Autodesk Inventor part; units mm, degrees
(part 3 of 6)
  line L900 (29.3831, -15.4753) -> (29.375, -15.3073) construction
  line L901 (29.375, -15.3073) -> (29.4167, -15.1213) construction
  line L902 (29.4167, -15.1213) -> (29.4167, -15.1153)
  spline S269 degree 3 poles (29.4167, -15.1153) (29.4167, -15.1093) (29.4252, -15.1093) (29.4252, -15.1034) knots 10 10 10 10 11 11 11 11
  line L903 (29.4167, -15.1153) -> (29.4167, -15.1093) construction
  line L904 (29.4167, -15.1093) -> (29.4252, -15.1093) construction
  line L905 (29.4252, -15.1093) -> (29.4252, -15.1034) construction
  line L906 (29.4252, -15.1034) -> (29.4149, -15.1093)
  spline S270 degree 3 poles (29.4149, -15.1093) (29.4209, -15.1034) (29.4167, -15.1034) (29.4167, -15.0974) knots 12 12 12 12 13 13 13 13
  line L907 (29.4149, -15.1093) -> (29.4209, -15.1034) construction
  line L908 (29.4209, -15.1034) -> (29.4167, -15.1034) construction
  line L909 (29.4167, -15.1034) -> (29.4167, -15.0974) construction
  line L910 (29.4167, -15.0974) -> (29.4167, -15.0673)
  spline S271 degree 3 poles (29.4167, -15.0673) (29.5, -14.7134) (29.6142, -14.3654) (29.7402, -14.0234) knots 14 14 14 14 15 15 15 15
  line L911 (29.4167, -15.0673) -> (29.5, -14.7134) construction
  line L912 (29.5, -14.7134) -> (29.6142, -14.3654) construction
  line L913 (29.6142, -14.3654) -> (29.7402, -14.0234) construction
  spline S272 degree 3 poles (29.7402, -14.0234) (29.8722, -13.6634) (30.0009, -13.3094) (30.1689, -12.9674) knots 15 15 15 15 16 16 16 16
  line L914 (29.7402, -14.0234) -> (29.8722, -13.6634) construction
  line L915 (29.8722, -13.6634) -> (30.0009, -13.3094) construction
  line L916 (30.0009, -13.3094) -> (30.1689, -12.9674) construction
  spline S273 degree 3 poles (30.1689, -12.9674) (30.3249, -12.6434) (30.5063, -12.3254) (30.7103, -12.0314) knots 16 16 16 16 17 17 17 17
  line L917 (30.1689, -12.9674) -> (30.3249, -12.6434) construction
  line L918 (30.3249, -12.6434) -> (30.5063, -12.3254) construction
  line L919 (30.5063, -12.3254) -> (30.7103, -12.0314) construction
  spline S274 degree 3 poles (30.7103, -12.0314) (30.8903, -11.7614) (31.1069, -11.4674) (31.3829, -11.2874) knots 17 17 17 17 18 18 18 18
  line L920 (30.7103, -12.0314) -> (30.8903, -11.7614) construction
  line L921 (30.8903, -11.7614) -> (31.1069, -11.4674) construction
  line L922 (31.1069, -11.4674) -> (31.3829, -11.2874) construction
  spline S275 degree 3 poles (31.3829, -11.2874) (31.467, -11.2634) (31.5513, -11.1734) (31.6593, -11.1914) knots 18 18 18 18 19 19 19 19
  line L923 (31.3829, -11.2874) -> (31.467, -11.2634) construction
  line L924 (31.467, -11.2634) -> (31.5513, -11.1734) construction
  line L925 (31.5513, -11.1734) -> (31.6593, -11.1914) construction
  spline S276 degree 3 poles (31.6593, -11.1914) (31.7673, -11.2094) (31.7675, -11.3234) (31.7435, -11.4314) knots 19 19 19 19 20 20 20 20
  line L926 (31.6593, -11.1914) -> (31.7673, -11.2094) construction
  line L927 (31.7673, -11.2094) -> (31.7675, -11.3234) construction
  line L928 (31.7675, -11.3234) -> (31.7435, -11.4314) construction
  spline S277 degree 3 poles (31.7435, -11.4314) (31.7735, -11.3474) (31.7915, -11.2574) (31.7196, -11.1974) knots 20 20 20 20 21 21 21 21
  line L929 (31.7435, -11.4314) -> (31.7735, -11.3474) construction
  line L930 (31.7735, -11.3474) -> (31.7915, -11.2574) construction
  line L931 (31.7915, -11.2574) -> (31.7196, -11.1974) construction
  spline S278 degree 3 poles (31.7196, -11.1974) (31.6235, -11.1254) (31.4376, -11.2394) (31.3596, -11.2934) knots 21 21 21 21 22 22 22 22
  line L932 (31.7196, -11.1974) -> (31.6235, -11.1254) construction
  line L933 (31.6235, -11.1254) -> (31.4376, -11.2394) construction
  line L934 (31.4376, -11.2394) -> (31.3596, -11.2934) construction
  spline S279 degree 3 poles (31.3596, -11.2934) (31.3236, -11.3054) (31.2876, -11.3294) (31.2576, -11.3534) knots 22 22 22 22 23 23 23 23
  line L935 (31.3596, -11.2934) -> (31.3236, -11.3054) construction
  line L936 (31.3236, -11.3054) -> (31.2876, -11.3294) construction
  line L937 (31.2876, -11.3294) -> (31.2576, -11.3534) construction
  spline S280 degree 3 poles (31.2576, -11.3534) (31.2756, -11.3354) (31.2996, -11.3174) (31.3296, -11.2994) knots 23 23 23 23 24 24 24 24
  line L938 (31.2576, -11.3534) -> (31.2756, -11.3354) construction
  line L939 (31.2756, -11.3354) -> (31.2996, -11.3174) construction
  line L940 (31.2996, -11.3174) -> (31.3296, -11.2994) construction
  line L941 (31.3296, -11.2994) -> (31.2996, -11.3114)
  line L942 (31.2996, -11.3114) -> (31.3836, -11.2634)
  spline S281 degree 3 poles (31.3836, -11.2634) (31.4797, -11.2094) (31.6956, -11.0894) (31.7676, -11.2454) knots 26 26 26 26 27 27 27 27
  line L943 (31.3836, -11.2634) -> (31.4797, -11.2094) construction
  line L944 (31.4797, -11.2094) -> (31.6956, -11.0894) construction
  line L945 (31.6956, -11.0894) -> (31.7676, -11.2454) construction
  spline S282 degree 3 poles (31.7676, -11.2454) (31.8216, -11.3714) (31.7376, -11.5814) (31.6956, -11.7014) knots 27 27 27 27 28 28 28 28
  line L946 (31.7676, -11.2454) -> (31.8216, -11.3714) construction
  line L947 (31.8216, -11.3714) -> (31.7376, -11.5814) construction
  line L948 (31.7376, -11.5814) -> (31.6956, -11.7014) construction
  spline S283 degree 3 poles (31.6956, -11.7014) (31.6176, -11.9054) (31.5216, -12.0974) (31.4196, -12.2894) knots 28 28 28 28 29 29 29 29
  line L949 (31.6956, -11.7014) -> (31.6176, -11.9054) construction
  line L950 (31.6176, -11.9054) -> (31.5216, -12.0974) construction
  line L951 (31.5216, -12.0974) -> (31.4196, -12.2894) construction
  spline S284 degree 3 poles (31.4196, -12.2894) (31.4376, -12.2474) (31.5096, -12.0887) (31.5096, -12.0885) knots 29 29 29 29 30 30 30 30
  line L952 (31.4196, -12.2894) -> (31.4376, -12.2474) construction
  line L953 (31.4376, -12.2474) -> (31.5096, -12.0885) construction
  line L954 (31.5096, -12.0885) -> (31.5096, -12.0885) construction
  spline S285 degree 3 poles (31.5096, -12.0885) (31.4677, -12.0825) (31.2756, -12.5417) (31.2396, -12.5417) knots 30 30 30 30 31 31 31 31
  line L955 (31.5096, -12.0885) -> (31.4677, -12.0825) construction
  line L956 (31.4677, -12.0825) -> (31.2756, -12.5417) construction
  line L957 (31.2756, -12.5417) -> (31.2396, -12.5417) construction
  line L958 (31.2396, -12.5417) -> (31.2456, -12.5417)
  spline S286 degree 3 poles (31.2456, -12.5417) (31.2216, -12.5417) (31.2037, -12.5745) (31.2037, -12.5805) knots 32 32 32 32 33 33 33 33
  line L959 (31.2456, -12.5417) -> (31.2216, -12.5417) construction
  line L960 (31.2216, -12.5417) -> (31.2037, -12.5745) construction
  line L961 (31.2037, -12.5745) -> (31.2037, -12.5805) construction
  spline S287 degree 3 poles (31.2037, -12.5805) (31.1917, -12.6525) (31.2756, -12.633) (31.3236, -12.627) knots 33 33 33 33 34 34 34 34
  line L962 (31.2037, -12.5805) -> (31.1917, -12.6525) construction
  line L963 (31.1917, -12.6525) -> (31.2756, -12.633) construction
  line L964 (31.2756, -12.633) -> (31.3236, -12.627) construction
  spline S288 degree 3 poles (31.3236, -12.627) (31.5276, -12.603) (31.7933, -12.4282) (31.9253, -12.2782) knots 34 34 34 34 35 35 35 35
  line L965 (31.3236, -12.627) -> (31.5276, -12.603) construction
  line L966 (31.5276, -12.603) -> (31.7933, -12.4282) construction
  line L967 (31.7933, -12.4282) -> (31.9253, -12.2782) construction
  spline S289 degree 3 poles (31.9253, -12.2782) (32.0693, -12.1162) (32.125, -11.8694) (32.125, -11.6534) knots 35 35 35 35 36 36 36 36
  line L968 (31.9253, -12.2782) -> (32.0693, -12.1162) construction
  line L969 (32.0693, -12.1162) -> (32.125, -11.8694) construction
  line L970 (32.125, -11.8694) -> (32.125, -11.6534) construction
  line L971 (32.125, -11.6534) -> (32.125, -11.6474)
  spline S290 degree 3 poles (32.125, -11.6474) (32.125, -11.2394) (31.8353, -10.7234) (31.3494, -10.7534) knots 37 37 37 37 38 38 38 38
  line L972 (32.125, -11.6474) -> (32.125, -11.2394) construction
  line L973 (32.125, -11.2394) -> (31.8353, -10.7234) construction
  line L974 (31.8353, -10.7234) -> (31.3494, -10.7534) construction
  spline S291 degree 3 poles (31.3494, -10.7534) (31.0793, -10.7654) (30.8265, -11.0294) (30.6525, -11.2094) knots 38 38 38 38 39 39 39 39
  line L975 (31.3494, -10.7534) -> (31.0793, -10.7654) construction
  line L976 (31.0793, -10.7654) -> (30.8265, -11.0294) construction
  line L977 (30.8265, -11.0294) -> (30.6525, -11.2094) construction
  spline S292 degree 3 poles (30.6525, -11.2094) (30.5265, -11.3534) (30.406, -11.5094) (30.2981, -11.6654) knots 39 39 39 39 40 40 40 40
  line L978 (30.6525, -11.2094) -> (30.5265, -11.3534) construction
  line L979 (30.5265, -11.3534) -> (30.406, -11.5094) construction
  line L980 (30.406, -11.5094) -> (30.2981, -11.6654) construction
  spline S293 degree 3 poles (30.2981, -11.6654) (30.2501, -11.7374) (30.2019, -11.8034) (30.1599, -11.8754) knots 40 40 40 40 41 41 41 41
  line L981 (30.2981, -11.6654) -> (30.2501, -11.7374) construction
  line L982 (30.2501, -11.7374) -> (30.2019, -11.8034) construction
  line L983 (30.2019, -11.8034) -> (30.1599, -11.8754) construction
  spline S294 degree 3 poles (30.1599, -11.8754) (30.1119, -11.9414) (30.0158, -12.0434) (29.9918, -12.1214) knots 41 41 41 41 42 42 42 42
  line L984 (30.1599, -11.8754) -> (30.1119, -11.9414) construction
  line L985 (30.1119, -11.9414) -> (30.0158, -12.0434) construction
  line L986 (30.0158, -12.0434) -> (29.9918, -12.1214) construction
  spline S295 degree 3 poles (29.9918, -12.1214) (29.9918, -12.1214) (30.0217, -12.0854) (30.0457, -12.0614) knots 42 42 42 42 43 43 43 43
  line L987 (29.9918, -12.1214) -> (29.9918, -12.1214) construction
  line L988 (29.9918, -12.1214) -> (30.0217, -12.0854) construction
  line L989 (30.0217, -12.0854) -> (30.0457, -12.0614) construction
  spline S296 degree 3 poles (30.0457, -12.0614) (29.9797, -12.1634) (29.9197, -12.2714) (29.8597, -12.3734) knots 43 43 43 43 44 44 44 44
  line L990 (30.0457, -12.0614) -> (29.9797, -12.1634) construction
  line L991 (29.9797, -12.1634) -> (29.9197, -12.2714) construction
  line L992 (29.9197, -12.2714) -> (29.8597, -12.3734) construction
  spline S297 degree 3 poles (29.8597, -12.3734) (29.8537, -12.3674) (29.8956, -12.2835) (29.8957, -12.2834) knots 44 44 44 44 45 45 45 45
  line L993 (29.8597, -12.3734) -> (29.8537, -12.3674) construction
  line L994 (29.8537, -12.3674) -> (29.8957, -12.2834) construction
  line L995 (29.8957, -12.2834) -> (29.8957, -12.2834) construction
  spline S298 degree 3 poles (29.8957, -12.2834) (29.8417, -12.2714) (29.5957, -12.7634) (29.5657, -12.8174) knots 45 45 45 45 46 46 46 46
  line L996 (29.8957, -12.2834) -> (29.8417, -12.2714) construction
  line L997 (29.8417, -12.2714) -> (29.5957, -12.7634) construction
  line L998 (29.5957, -12.7634) -> (29.5657, -12.8174) construction
  spline S299 degree 3 poles (29.5657, -12.8174) (29.4577, -13.0154) (29.3617, -13.2134) (29.2957, -13.4234) knots 46 46 46 46 47 47 47 47
  line L999 (29.5657, -12.8174) -> (29.4577, -13.0154) construction
  line L1000 (29.4577, -13.0154) -> (29.3617, -13.2134) construction
  line L1001 (29.3617, -13.2134) -> (29.2957, -13.4234) construction
  spline S300 degree 3 poles (29.2957, -13.4234) (29.2237, -13.6574) (29.1277, -13.8794) (29.0557, -14.1074) knots 47 47 47 47 48 48 48 48
  line L1002 (29.2957, -13.4234) -> (29.2237, -13.6574) construction
  line L1003 (29.2237, -13.6574) -> (29.1277, -13.8794) construction
  line L1004 (29.1277, -13.8794) -> (29.0557, -14.1074) construction
  spline S301 degree 3 poles (29.0557, -14.1074) (29.0197, -14.2214) (28.9837, -14.3294) (28.9597, -14.4434) knots 48 48 48 48 49 49 49 49
  line L1005 (29.0557, -14.1074) -> (29.0197, -14.2214) construction
  line L1006 (29.0197, -14.2214) -> (28.9837, -14.3294) construction
  line L1007 (28.9837, -14.3294) -> (28.9597, -14.4434) construction
  spline S302 degree 3 poles (28.9597, -14.4434) (28.9477, -14.4974) (28.9357, -14.5453) (28.9297, -14.5993) knots 49 49 49 49 50 50 50 50
  line L1008 (28.9597, -14.4434) -> (28.9477, -14.4974) construction
  line L1009 (28.9477, -14.4974) -> (28.9357, -14.5453) construction
  line L1010 (28.9357, -14.5453) -> (28.9297, -14.5993) construction
  spline S303 degree 3 poles (28.9297, -14.5993) (28.9297, -14.6053) (28.9177, -14.7014) (28.9297, -14.6894) knots 50 50 50 50 51 51 51 51
  line L1011 (28.9297, -14.5993) -> (28.9297, -14.6053) construction
  line L1012 (28.9297, -14.6053) -> (28.9177, -14.7014) construction
  line L1013 (28.9177, -14.7014) -> (28.9297, -14.6894) construction
  spline S304 degree 3 poles (28.9297, -14.6894) (28.9177, -14.7313) (28.9177, -14.7853) (28.9117, -14.8274) knots 51 51 51 51 52 52 52 52
  line L1014 (28.9297, -14.6894) -> (28.9177, -14.7313) construction
  line L1015 (28.9177, -14.7313) -> (28.9177, -14.7853) construction
  line L1016 (28.9177, -14.7853) -> (28.9117, -14.8274) construction
  spline S305 degree 3 poles (28.9117, -14.8274) (28.9117, -14.8272) (28.9117, -14.7253) (28.9177, -14.7134) knots 52 52 52 52 53 53 53 53
  line L1017 (28.9117, -14.8274) -> (28.9117, -14.8274) construction
  line L1018 (28.9117, -14.8274) -> (28.9117, -14.7253) construction
  line L1019 (28.9117, -14.7253) -> (28.9177, -14.7134) construction
  spline S306 degree 3 poles (28.9177, -14.7134) (28.8937, -14.7433) (28.9117, -14.8573) (28.9057, -14.8693) knots 53 53 53 53 54 54 54 54
  line L1020 (28.9177, -14.7134) -> (28.8937, -14.7433) construction
  line L1021 (28.8937, -14.7433) -> (28.9117, -14.8573) construction
  line L1022 (28.9117, -14.8573) -> (28.9057, -14.8693) construction
  spline S307 degree 3 poles (28.9057, -14.8693) (28.8757, -15.0974) (28.8277, -15.3373) (28.9057, -15.5593) knots 54 54 54 54 55 55 55 55
  line L1023 (28.9057, -14.8693) -> (28.8757, -15.0974) construction
  line L1024 (28.8757, -15.0974) -> (28.8277, -15.3373) construction
  line L1025 (28.8277, -15.3373) -> (28.9057, -15.5593) construction
  spline S308 degree 3 poles (28.9057, -15.5593) (29.0077, -15.8653) (29.2597, -16.1173) (29.5357, -16.2793) knots 55 55 55 55 56 56 56 56
  line L1026 (28.9057, -15.5593) -> (29.0077, -15.8653) construction
  line L1027 (29.0077, -15.8653) -> (29.2597, -16.1173) construction
  line L1028 (29.2597, -16.1173) -> (29.5357, -16.2793) construction
  spline S309 degree 3 poles (29.5357, -16.2793) (29.6797, -16.3693) (29.8717, -16.4713) (30.0517, -16.4593) knots 56 56 56 56 57 57 57 57
  line L1029 (29.5357, -16.2793) -> (29.6797, -16.3693) construction
  line L1030 (29.6797, -16.3693) -> (29.8717, -16.4713) construction
  line L1031 (29.8717, -16.4713) -> (30.0517, -16.4593) construction
  spline S310 degree 3 poles (30.0517, -16.4593) (30.2617, -16.4473) (30.4657, -16.2733) (30.6217, -16.1473) knots 57 57 57 57 58 58 58 58
  line L1032 (30.0517, -16.4593) -> (30.2617, -16.4473) construction
  line L1033 (30.2617, -16.4473) -> (30.4657, -16.2733) construction
  line L1034 (30.4657, -16.2733) -> (30.6217, -16.1473) construction
  spline S311 degree 3 poles (30.6217, -16.1473) (31.0776, -15.7633) (31.4916, -15.2233) (31.5696, -14.6113) knots 58 58 58 58 59 59 59 59
  line L1035 (30.6217, -16.1473) -> (31.0776, -15.7633) construction
  line L1036 (31.0776, -15.7633) -> (31.4916, -15.2233) construction
  line L1037 (31.4916, -15.2233) -> (31.5696, -14.6113) construction
  spline S312 degree 3 poles (31.5696, -14.6113) (31.5756, -14.5694) (31.6056, -14.3594) (31.5337, -14.3534) knots 59 59 59 59 60 60 60 60
  line L1038 (31.5696, -14.6113) -> (31.5756, -14.5694) construction
  line L1039 (31.5756, -14.5694) -> (31.6056, -14.3594) construction
  line L1040 (31.6056, -14.3594) -> (31.5337, -14.3534) construction
  spline S313 degree 3 poles (31.7076, -11.5814) (31.7136, -11.5694) (31.7136, -11.5634) (31.7136, -11.5574) (31.7256, -11.5214) (31.7376, -11.4794) (31.7437, -11.4314) (31.7316, -11.4854) (31.7076, -11.5394) (31.7076, -11.5814) knots 0 0 0 0 1 1 1 2 2 2 3 3 3 3
  line L1041 (31.7076, -11.5814) -> (31.7136, -11.5694) construction
  line L1042 (31.7136, -11.5694) -> (31.7136, -11.5634) construction
  line L1043 (31.7136, -11.5634) -> (31.7136, -11.5574) construction
  line L1044 (31.7136, -11.5574) -> (31.7256, -11.5214) construction
  line L1045 (31.7256, -11.5214) -> (31.7376, -11.4794) construction
  line L1046 (31.7376, -11.4794) -> (31.7437, -11.4314) construction
  line L1047 (31.7437, -11.4314) -> (31.7316, -11.4854) construction
  line L1048 (31.7316, -11.4854) -> (31.7076, -11.5394) construction
  line L1049 (31.7076, -11.5394) -> (31.7076, -11.5814) construction
  spline S314 degree 3 poles (27.3997, -14.1434) (27.3277, -14.1974) (27.2977, -14.2814) (27.2437, -14.3413) knots 0 0 0 0 1 1 1 1
  line L1050 (27.3997, -14.1434) -> (27.3277, -14.1974) construction
  line L1051 (27.3277, -14.1974) -> (27.2977, -14.2814) construction
  line L1052 (27.2977, -14.2814) -> (27.2437, -14.3413) construction
  spline S315 degree 3 poles (27.2437, -14.3413) (27.1537, -14.4434) (27.0337, -14.5333) (26.9137, -14.5933) knots 1 1 1 1 2 2 2 2
  line L1053 (27.2437, -14.3413) -> (27.1537, -14.4434) construction
  line L1054 (27.1537, -14.4434) -> (27.0337, -14.5333) construction
  line L1055 (27.0337, -14.5333) -> (26.9137, -14.5933) construction
  spline S316 degree 3 poles (26.9137, -14.5933) (26.8477, -14.6174) (26.7997, -14.6713) (26.7517, -14.6954) knots 2 2 2 2 3 3 3 3
  line L1056 (26.9137, -14.5933) -> (26.8477, -14.6174) construction
  line L1057 (26.8477, -14.6174) -> (26.7997, -14.6713) construction
  line L1058 (26.7997, -14.6713) -> (26.7517, -14.6954) construction
  spline S317 degree 3 poles (26.7517, -14.6954) (26.6857, -14.7433) (26.5837, -14.7253) (26.5117, -14.7253) knots 3 3 3 3 4 4 4 4
  line L1059 (26.7517, -14.6954) -> (26.6857, -14.7433) construction
  line L1060 (26.6857, -14.7433) -> (26.5837, -14.7253) construction
  line L1061 (26.5837, -14.7253) -> (26.5117, -14.7253) construction
  spline S318 degree 3 poles (26.5117, -14.7253) (26.6017, -14.5034) (26.6617, -14.2634) (26.7937, -14.0654) knots 4 4 4 4 5 5 5 5
  line L1062 (26.5117, -14.7253) -> (26.6017, -14.5034) construction
  line L1063 (26.6017, -14.5034) -> (26.6617, -14.2634) construction
  line L1064 (26.6617, -14.2634) -> (26.7937, -14.0654) construction
  spline S319 degree 3 poles (26.7937, -14.0654) (26.8537, -13.9874) (26.9257, -13.8974) (26.8957, -13.7894) knots 5 5 5 5 6 6 6 6
  line L1065 (26.7937, -14.0654) -> (26.8537, -13.9874) construction
  line L1066 (26.8537, -13.9874) -> (26.9257, -13.8974) construction
  line L1067 (26.9257, -13.8974) -> (26.8957, -13.7894) construction
  spline S320 degree 3 poles (26.8957, -13.7894) (26.8717, -13.7174) (26.7997, -13.6634) (26.7277, -13.6934) knots 6 6 6 6 7 7 7 7
  line L1068 (26.8957, -13.7894) -> (26.8717, -13.7174) construction
  line L1069 (26.8717, -13.7174) -> (26.7997, -13.6634) construction
  line L1070 (26.7997, -13.6634) -> (26.7277, -13.6934) construction
  spline S321 degree 3 poles (26.7277, -13.6934) (26.7097, -13.6994) (26.7037, -13.7174) (26.6857, -13.7294) knots 7 7 7 7 8 8 8 8
  line L1071 (26.7277, -13.6934) -> (26.7097, -13.6994) construction
  line L1072 (26.7097, -13.6994) -> (26.7037, -13.7174) construction
  line L1073 (26.7037, -13.7174) -> (26.6857, -13.7294) construction
  spline S322 degree 3 poles (26.6857, -13.7294) (26.5837, -13.8254) (26.4697, -13.9454) (26.3917, -14.0654) knots 8 8 8 8 9 9 9 9
  line L1074 (26.6857, -13.7294) -> (26.5837, -13.8254) construction
  line L1075 (26.5837, -13.8254) -> (26.4697, -13.9454) construction
  line L1076 (26.4697, -13.9454) -> (26.3917, -14.0654) construction
  spline S323 degree 3 poles (26.3917, -14.0654) (26.3197, -14.1794) (26.2717, -14.2994) (26.2417, -14.4314) knots 9 9 9 9 10 10 10 10
  line L1077 (26.3917, -14.0654) -> (26.3197, -14.1794) construction
  line L1078 (26.3197, -14.1794) -> (26.2717, -14.2994) construction
  line L1079 (26.2717, -14.2994) -> (26.2417, -14.4314) construction
  spline S324 degree 3 poles (26.2417, -14.4314) (26.2357, -14.4554) (26.2297, -14.7674) (26.2237, -14.7674) knots 10 10 10 10 11 11 11 11
  line L1080 (26.2417, -14.4314) -> (26.2357, -14.4554) construction
  line L1081 (26.2357, -14.4554) -> (26.2297, -14.7674) construction
  line L1082 (26.2297, -14.7674) -> (26.2237, -14.7674) construction
  line L1083 (26.2237, -14.7674) -> (26.2477, -14.7493)
  spline S325 degree 3 poles (26.2477, -14.7493) (26.2537, -14.7853) (26.1277, -14.9473) (26.0977, -14.9953) knots 12 12 12 12 13 13 13 13
  line L1084 (26.2477, -14.7493) -> (26.2537, -14.7853) construction
  line L1085 (26.2537, -14.7853) -> (26.1277, -14.9473) construction
  line L1086 (26.1277, -14.9473) -> (26.0977, -14.9953) construction
  spline S326 degree 3 poles (26.0977, -14.9953) (26.0317, -15.1153) (25.9657, -15.2353) (25.8937, -15.3553) knots 13 13 13 13 14 14 14 14
  line L1087 (26.0977, -14.9953) -> (26.0317, -15.1153) construction
  line L1088 (26.0317, -15.1153) -> (25.9657, -15.2353) construction
  line L1089 (25.9657, -15.2353) -> (25.8937, -15.3553) construction
  spline S327 degree 3 poles (25.8937, -15.3553) (25.8337, -15.4573) (25.6597, -15.8773) (25.5157, -15.8593) knots 14 14 14 14 15 15 15 15
  line L1090 (25.8937, -15.3553) -> (25.8337, -15.4573) construction
  line L1091 (25.8337, -15.4573) -> (25.6597, -15.8773) construction
  line L1092 (25.6597, -15.8773) -> (25.5157, -15.8593) construction
  spline S328 degree 3 poles (25.5157, -15.8593) (25.2097, -15.8293) (25.6237, -14.5694) (25.6117, -14.5634) knots 15 15 15 15 16 16 16 16
  line L1093 (25.5157, -15.8593) -> (25.2097, -15.8293) construction
  line L1094 (25.2097, -15.8293) -> (25.6237, -14.5694) construction
  line L1095 (25.6237, -14.5694) -> (25.6117, -14.5634) construction
  spline S329 degree 3 poles (25.6117, -14.5634) (25.5817, -14.5574) (25.4497, -15.1453) (25.4317, -15.2473) knots 16 16 16 16 17 17 17 17
  line L1096 (25.6117, -14.5634) -> (25.5817, -14.5574) construction
  line L1097 (25.5817, -14.5574) -> (25.4497, -15.1453) construction
  line L1098 (25.4497, -15.1453) -> (25.4317, -15.2473) construction
  spline S330 degree 3 poles (25.4317, -15.2473) (25.4857, -14.9054) (25.5757, -14.5634) (25.6897, -14.2394) knots 17 17 17 17 18 18 18 18
  line L1099 (25.4317, -15.2473) -> (25.4857, -14.9054) construction
  line L1100 (25.4857, -14.9054) -> (25.5757, -14.5634) construction
  line L1101 (25.5757, -14.5634) -> (25.6897, -14.2394) construction
  spline S331 degree 3 poles (25.6897, -14.2394) (25.6837, -14.2694) (25.6717, -14.3174) (25.6777, -14.3174) knots 18 18 18 18 19 19 19 19
  line L1102 (25.6897, -14.2394) -> (25.6837, -14.2694) construction
  line L1103 (25.6837, -14.2694) -> (25.6717, -14.3174) construction
  line L1104 (25.6717, -14.3174) -> (25.6777, -14.3174) construction
  spline S332 degree 3 poles (25.6777, -14.3174) (25.7017, -14.3234) (25.7797, -14.0894) (25.7677, -14.0894) knots 19 19 19 19 20 20 20 20
  line L1105 (25.6777, -14.3174) -> (25.7017, -14.3234) construction
  line L1106 (25.7017, -14.3234) -> (25.7797, -14.0894) construction
  line L1107 (25.7797, -14.0894) -> (25.7677, -14.0894) construction
  line L1108 (25.7677, -14.0894) -> (25.7377, -14.1074)
  spline S333 degree 3 poles (25.7377, -14.1074) (25.7557, -14.0774) (25.7977, -14.0654) (25.8037, -14.0234) knots 21 21 21 21 22 22 22 22
  line L1109 (25.7377, -14.1074) -> (25.7557, -14.0774) construction
  line L1110 (25.7557, -14.0774) -> (25.7977, -14.0654) construction
  line L1111 (25.7977, -14.0654) -> (25.8037, -14.0234) construction
  spline S334 degree 3 poles (25.8037, -14.0234) (25.8157, -13.9514) (25.7677, -13.8974) (25.7137, -13.8614) knots 22 22 22 22 23 23 23 23
  line L1112 (25.8037, -14.0234) -> (25.8157, -13.9514) construction
  line L1113 (25.8157, -13.9514) -> (25.7677, -13.8974) construction
  line L1114 (25.7677, -13.8974) -> (25.7137, -13.8614) construction
  spline S335 degree 3 poles (25.7137, -13.8614) (25.5877, -13.7714) (25.4197, -13.8254) (25.3237, -13.9334) knots 23 23 23 23 24 24 24 24
  line L1115 (25.7137, -13.8614) -> (25.5877, -13.7714) construction
  line L1116 (25.5877, -13.7714) -> (25.4197, -13.8254) construction
  line L1117 (25.4197, -13.8254) -> (25.3237, -13.9334) construction
  spline S336 degree 3 poles (25.3237, -13.9334) (25.2517, -14.0234) (25.1917, -14.1374) (25.1257, -14.2334) knots 24 24 24 24 25 25 25 25
  line L1118 (25.3237, -13.9334) -> (25.2517, -14.0234) construction
  line L1119 (25.2517, -14.0234) -> (25.1917, -14.1374) construction
  line L1120 (25.1917, -14.1374) -> (25.1257, -14.2334) construction
  spline S337 degree 3 poles (25.1257, -14.2334) (25.0657, -14.3174) (25.0057, -14.3954) (24.9517, -14.4793) knots 25 25 25 25 26 26 26 26
  line L1121 (25.1257, -14.2334) -> (25.0657, -14.3174) construction
  line L1122 (25.0657, -14.3174) -> (25.0057, -14.3954) construction
  line L1123 (25.0057, -14.3954) -> (24.9517, -14.4793) construction
  spline S338 degree 3 poles (24.9517, -14.4793) (24.9337, -14.5034) (24.7897, -14.7253) (24.8017, -14.7253) knots 26 26 26 26 27 27 27 27
  line L1124 (24.9517, -14.4793) -> (24.9337, -14.5034) construction
  line L1125 (24.9337, -14.5034) -> (24.7897, -14.7253) construction
  line L1126 (24.7897, -14.7253) -> (24.8017, -14.7253) construction
  spline S339 degree 3 poles (24.8017, -14.7253) (24.8137, -14.7194) (24.8257, -14.7134) (24.8377, -14.7014) knots 27 27 27 27 28 28 28 28
  line L1127 (24.8017, -14.7253) -> (24.8137, -14.7194) construction
  line L1128 (24.8137, -14.7194) -> (24.8257, -14.7134) construction
  line L1129 (24.8257, -14.7134) -> (24.8377, -14.7014) construction
  spline S340 degree 3 poles (24.8377, -14.7014) (24.7237, -14.8513) (24.5497, -15.0253) (24.4057, -15.1634) knots 28 28 28 28 29 29 29 29
  line L1130 (24.8377, -14.7014) -> (24.7237, -14.8513) construction
  line L1131 (24.7237, -14.8513) -> (24.5497, -15.0253) construction
  line L1132 (24.5497, -15.0253) -> (24.4057, -15.1634) construction
  spline S341 degree 3 poles (24.4057, -15.1634) (24.3457, -15.2173) (24.2017, -15.3973) (24.1058, -15.3793) knots 29 29 29 29 30 30 30 30
  line L1133 (24.4057, -15.1634) -> (24.3457, -15.2173) construction
  line L1134 (24.3457, -15.2173) -> (24.2017, -15.3973) construction
  line L1135 (24.2017, -15.3973) -> (24.1058, -15.3793) construction
  spline S342 degree 3 poles (24.1058, -15.3793) (23.8058, -15.3253) (24.3937, -14.1254) (24.3818, -14.1194) knots 30 30 30 30 31 31 31 31
  line L1136 (24.1058, -15.3793) -> (23.8058, -15.3253) construction
  line L1137 (23.8058, -15.3253) -> (24.3937, -14.1254) construction
  line L1138 (24.3937, -14.1254) -> (24.3818, -14.1194) construction
  spline S343 degree 3 poles (24.3818, -14.1194) (24.3637, -14.1134) (24.1477, -14.6593) (24.1298, -14.7014) knots 31 31 31 31 32 32 32 32
  line L1139 (24.3818, -14.1194) -> (24.3637, -14.1134) construction
  line L1140 (24.3637, -14.1134) -> (24.1477, -14.6593) construction
  line L1141 (24.1477, -14.6593) -> (24.1298, -14.7014) construction
  spline S344 degree 3 poles (24.1298, -14.7014) (24.2318, -14.4013) (24.3637, -14.1134) (24.4957, -13.8254) knots 32 32 32 32 33 33 33 33
  line L1142 (24.1298, -14.7014) -> (24.2318, -14.4013) construction
  line L1143 (24.2318, -14.4013) -> (24.3637, -14.1134) construction
  line L1144 (24.3637, -14.1134) -> (24.4957, -13.8254) construction
  spline S345 degree 3 poles (24.4957, -13.8254) (24.5017, -13.8254) (24.4657, -13.9154) (24.4717, -13.9154) knots 33 33 33 33 34 34 34 34
  line L1145 (24.4957, -13.8254) -> (24.5017, -13.8254) construction
  line L1146 (24.5017, -13.8254) -> (24.4657, -13.9154) construction
  line L1147 (24.4657, -13.9154) -> (24.4717, -13.9154) construction
  spline S346 degree 3 poles (24.4717, -13.9154) (24.4897, -13.9214) (24.5857, -13.7234) (24.5617, -13.7174) knots 34 34 34 34 35 35 35 35
  line L1148 (24.4717, -13.9154) -> (24.4897, -13.9214) construction
  line L1149 (24.4897, -13.9214) -> (24.5857, -13.7234) construction
  line L1150 (24.5857, -13.7234) -> (24.5617, -13.7174) construction
  line L1151 (24.5617, -13.7174) -> (24.5437, -13.7354)
  spline S347 degree 3 poles (24.5437, -13.7354) (24.5617, -13.7054) (24.5917, -13.6994) (24.5977, -13.6634) knots 36 36 36 36 37 37 37 37
  line L1152 (24.5437, -13.7354) -> (24.5617, -13.7054) construction
  line L1153 (24.5617, -13.7054) -> (24.5917, -13.6994) construction
  line L1154 (24.5917, -13.6994) -> (24.5977, -13.6634) construction
  spline S348 degree 3 poles (24.5977, -13.6634) (24.6157, -13.5914) (24.5617, -13.5254) (24.5078, -13.4894) knots 37 37 37 37 38 38 38 38
  line L1155 (24.5977, -13.6634) -> (24.6157, -13.5914) construction
  line L1156 (24.6157, -13.5914) -> (24.5617, -13.5254) construction
  line L1157 (24.5617, -13.5254) -> (24.5078, -13.4894) construction
  spline S349 degree 3 poles (24.5078, -13.4894) (24.3698, -13.3994) (24.1718, -13.4714) (24.0998, -13.6094) knots 38 38 38 38 39 39 39 39
  line L1158 (24.5078, -13.4894) -> (24.3698, -13.3994) construction
  line L1159 (24.3698, -13.3994) -> (24.1718, -13.4714) construction
  line L1160 (24.1718, -13.4714) -> (24.0998, -13.6094) construction
  spline S350 degree 3 poles (24.0998, -13.6094) (24.0817, -13.6394) (24.0877, -13.6754) (24.0578, -13.7054) knots 39 39 39 39 40 40 40 40
  line L1161 (24.0998, -13.6094) -> (24.0817, -13.6394) construction
  line L1162 (24.0817, -13.6394) -> (24.0877, -13.6754) construction
  line L1163 (24.0877, -13.6754) -> (24.0578, -13.7054) construction
  spline S351 degree 3 poles (24.0578, -13.7054) (24.0458, -13.7234) (23.9978, -13.7414) (23.9738, -13.7834) knots 40 40 40 40 41 41 41 41
  line L1164 (24.0578, -13.7054) -> (24.0458, -13.7234) construction
  line L1165 (24.0458, -13.7234) -> (23.9978, -13.7414) construction
  line L1166 (23.9978, -13.7414) -> (23.9738, -13.7834) construction
  spline S352 degree 3 poles (23.9738, -13.7834) (23.9205, -13.8706) (23.8867, -13.9734) (23.8536, -14.0729) knots 41 41 41 41 42 42 42 42
  line L1167 (23.9738, -13.7834) -> (23.9205, -13.8706) construction
  line L1168 (23.9205, -13.8706) -> (23.8867, -13.9734) construction
  line L1169 (23.8867, -13.9734) -> (23.8536, -14.0729) construction
  spline S353 degree 3 poles (23.8536, -14.0729) (23.8438, -14.0766) (23.8338, -14.0805) (23.8238, -14.0834) knots 42 42 42 42 43 43 43 43
  line L1170 (23.8536, -14.0729) -> (23.8438, -14.0766) construction
  line L1171 (23.8438, -14.0766) -> (23.8338, -14.0805) construction
  line L1172 (23.8338, -14.0805) -> (23.8238, -14.0834) construction
  spline S354 degree 3 poles (23.8238, -14.0834) (23.6498, -14.1194) (23.4698, -14.1614) (23.2898, -14.1914) knots 43 43 43 43 44 44 44 44
  line L1173 (23.8238, -14.0834) -> (23.6498, -14.1194) construction
  line L1174 (23.6498, -14.1194) -> (23.4698, -14.1614) construction
  line L1175 (23.4698, -14.1614) -> (23.2898, -14.1914) construction
  spline S355 degree 3 poles (23.2898, -14.1914) (23.3558, -13.9754) (23.4218, -13.7474) (23.4458, -13.5254) knots 44 44 44 44 45 45 45 45
  line L1176 (23.2898, -14.1914) -> (23.3558, -13.9754) construction
  line L1177 (23.3558, -13.9754) -> (23.4218, -13.7474) construction
  line L1178 (23.4218, -13.7474) -> (23.4458, -13.5254) construction
  spline S356 degree 3 poles (23.4458, -13.5254) (23.4578, -13.4414) (23.4638, -13.3514) (23.4458, -13.2674) knots 45 45 45 45 46 46 46 46
  line L1179 (23.4458, -13.5254) -> (23.4578, -13.4414) construction
  line L1180 (23.4578, -13.4414) -> (23.4638, -13.3514) construction
  line L1181 (23.4638, -13.3514) -> (23.4458, -13.2674) construction
  spline S357 degree 3 poles (23.4458, -13.2674) (23.4338, -13.2134) (23.4158, -13.1594) (23.3858, -13.1114) knots 46 46 46 46 47 47 47 47
  line L1182 (23.4458, -13.2674) -> (23.4338, -13.2134) construction
  line L1183 (23.4338, -13.2134) -> (23.4158, -13.1594) construction
  line L1184 (23.4158, -13.1594) -> (23.3858, -13.1114) construction
  spline S358 degree 3 poles (23.3858, -13.1114) (23.3857, -13.1113) (23.3138, -13.0214) (23.3318, -13.0694) knots 47 47 47 47 48 48 48 48
  line L1185 (23.3858, -13.1114) -> (23.3858, -13.1114) construction
  line L1186 (23.3858, -13.1114) -> (23.3138, -13.0214) construction
  line L1187 (23.3138, -13.0214) -> (23.3318, -13.0694) construction
  line L1188 (23.3318, -13.0694) -> (23.3258, -13.0634)
  line L1189 (23.3258, -13.0634) -> (23.3018, -13.0154)
  line L1190 (23.3018, -13.0154) -> (23.3258, -13.0394)
  spline S359 degree 3 poles (23.3258, -13.0394) (23.3318, -13.0034) (23.2299, -12.9374) (23.2298, -12.9374) knots 51 51 51 51 52 52 52 52
  line L1191 (23.3258, -13.0394) -> (23.3318, -13.0034) construction
  line L1192 (23.3318, -13.0034) -> (23.2298, -12.9374) construction
  line L1193 (23.2298, -12.9374) -> (23.2298, -12.9374) construction
  spline S360 degree 3 poles (23.2298, -12.9374) (23.0798, -12.7874) (22.8758, -12.6734) (22.6718, -12.7874) knots 52 52 52 52 53 53 53 53
  line L1194 (23.2298, -12.9374) -> (23.0798, -12.7874) construction
  line L1195 (23.0798, -12.7874) -> (22.8758, -12.6734) construction
  line L1196 (22.8758, -12.6734) -> (22.6718, -12.7874) construction
  spline S361 degree 3 poles (22.6718, -12.7874) (22.5458, -12.8594) (22.4438, -12.9794) (22.3598, -13.0994) knots 53 53 53 53 54 54 54 54
  line L1197 (22.6718, -12.7874) -> (22.5458, -12.8594) construction
  line L1198 (22.5458, -12.8594) -> (22.4438, -12.9794) construction
  line L1199 (22.4438, -12.9794) -> (22.3598, -13.0994) construction
  spline S362 degree 3 poles (22.3598, -13.0994) (22.3298, -13.1414) (22.2998, -13.1894) (22.2758, -13.2374) knots 54 54 54 54 55 55 55 55
  line L1200 (22.3598, -13.0994) -> (22.3298, -13.1414) construction
  line L1201 (22.3298, -13.1414) -> (22.2998, -13.1894) construction
  line L1202 (22.2998, -13.1894) -> (22.2758, -13.2374) construction
  spline S363 degree 3 poles (22.2758, -13.2374) (22.2518, -13.2854) (22.2158, -13.4414) (22.1798, -13.4654) knots 55 55 55 55 56 56 56 56
  line L1203 (22.2758, -13.2374) -> (22.2518, -13.2854) construction
  line L1204 (22.2518, -13.2854) -> (22.2158, -13.4414) construction
  line L1205 (22.2158, -13.4414) -> (22.1798, -13.4654) construction
  spline S364 degree 3 poles (22.1798, -13.4654) (22.1498, -13.4894) (22.0598, -13.4954) (22.0178, -13.5194) knots 56 56 56 56 57 57 57 57
  line L1206 (22.1798, -13.4654) -> (22.1498, -13.4894) construction
  line L1207 (22.1498, -13.4894) -> (22.0598, -13.4954) construction
  line L1208 (22.0598, -13.4954) -> (22.0178, -13.5194) construction
  spline S365 degree 3 poles (22.0178, -13.5194) (21.9578, -13.5434) (21.9038, -13.5734) (21.8558, -13.6094) knots 57 57 57 57 58 58 58 58
  line L1209 (22.0178, -13.5194) -> (21.9578, -13.5434) construction
  line L1210 (21.9578, -13.5434) -> (21.9038, -13.5734) construction
  line L1211 (21.9038, -13.5734) -> (21.8558, -13.6094) construction
  spline S366 degree 3 poles (21.8558, -13.6094) (21.7418, -13.6814) (21.6518, -13.7834) (21.5678, -13.8854) knots 58 58 58 58 59 59 59 59
  line L1212 (21.8558, -13.6094) -> (21.7418, -13.6814) construction
  line L1213 (21.7418, -13.6814) -> (21.6518, -13.7834) construction
  line L1214 (21.6518, -13.7834) -> (21.5678, -13.8854) construction
  spline S367 degree 3 poles (21.5678, -13.8854) (21.5301, -13.9356) (21.4975, -13.9875) (21.4679, -14.0402) knots 59 59 59 59 60 60 60 60
  line L1215 (21.5678, -13.8854) -> (21.5301, -13.9356) construction
  line L1216 (21.5301, -13.9356) -> (21.4975, -13.9875) construction
  line L1217 (21.4975, -13.9875) -> (21.4679, -14.0402) construction
  spline S368 degree 3 poles (21.4679, -14.0402) (21.4633, -14.0445) (21.4588, -14.0482) (21.4538, -14.0534) knots 60 60 60 60 61 61 61 61
  line L1218 (21.4679, -14.0402) -> (21.4633, -14.0445) construction
  line L1219 (21.4633, -14.0445) -> (21.4588, -14.0482) construction
  line L1220 (21.4588, -14.0482) -> (21.4538, -14.0534) construction
  spline S369 degree 3 poles (21.4538, -14.0534) (21.3698, -14.1434) (21.3158, -14.2934) (21.2498, -14.4013) knots 61 61 61 61 62 62 62 62
  line L1221 (21.4538, -14.0534) -> (21.3698, -14.1434) construction
  line L1222 (21.3698, -14.1434) -> (21.3158, -14.2934) construction
  line L1223 (21.3158, -14.2934) -> (21.2498, -14.4013) construction
  spline S370 degree 3 poles (21.2498, -14.4013) (21.1478, -14.5754) (21.0458, -14.7433) (20.9378, -14.9113) knots 62 62 62 62 63 63 63 63
  line L1224 (21.2498, -14.4013) -> (21.1478, -14.5754) construction
  line L1225 (21.1478, -14.5754) -> (21.0458, -14.7433) construction
  line L1226 (21.0458, -14.7433) -> (20.9378, -14.9113) construction
  spline S371 degree 3 poles (20.9378, -14.9113) (20.7338, -15.2353) (20.5298, -15.5653) (20.2839, -15.8593) knots 63 63 63 63 64 64 64 64
  line L1227 (20.9378, -14.9113) -> (20.7338, -15.2353) construction
  line L1228 (20.7338, -15.2353) -> (20.5298, -15.5653) construction
  line L1229 (20.5298, -15.5653) -> (20.2839, -15.8593) construction
  spline S372 degree 3 poles (20.2839, -15.8593) (20.1818, -15.9853) (19.9659, -16.2913) (19.7619, -16.2673) knots 64 64 64 64 65 65 65 65
  line L1230 (20.2839, -15.8593) -> (20.1818, -15.9853) construction
  line L1231 (20.1818, -15.9853) -> (19.9659, -16.2913) construction
  line L1232 (19.9659, -16.2913) -> (19.7619, -16.2673) construction
  spline S373 degree 3 poles (19.7619, -16.2673) (19.6119, -16.2433) (19.6119, -15.9853) (19.6119, -15.8713) (19.6119, -15.7753) (19.6179, -15.6793) (19.6299, -15.5893) knots 65 65 65 65 66 66 66 67 67 67 67
  line L1233 (19.7619, -16.2673) -> (19.6119, -16.2433) construction
  line L1234 (19.6119, -16.2433) -> (19.6119, -15.9853) construction
  line L1235 (19.6119, -15.9853) -> (19.6119, -15.8713) construction
  line L1236 (19.6119, -15.8713) -> (19.6119, -15.7753) construction
  line L1237 (19.6119, -15.7753) -> (19.6179, -15.6793) construction
  line L1238 (19.6179, -15.6793) -> (19.6299, -15.5893) construction
  spline S374 degree 3 poles (19.6299, -15.5893) (19.6359, -15.5353) (19.6839, -15.3553) (19.6539, -15.3073) knots 67 67 67 67 68 68 68 68
  line L1239 (19.6299, -15.5893) -> (19.6359, -15.5353) construction
  line L1240 (19.6359, -15.5353) -> (19.6839, -15.3553) construction
  line L1241 (19.6839, -15.3553) -> (19.6539, -15.3073) construction
  line L1242 (19.6539, -15.3073) -> (19.6059, -15.4873)
  spline S375 degree 3 poles (19.6059, -15.4873) (19.6119, -15.4153) (19.6239, -15.3373) (19.6419, -15.2653) knots 69 69 69 69 70 70 70 70
  line L1243 (19.6059, -15.4873) -> (19.6119, -15.4153) construction
  line L1244 (19.6119, -15.4153) -> (19.6239, -15.3373) construction
  line L1245 (19.6239, -15.3373) -> (19.6419, -15.2653) construction
  spline S376 degree 3 poles (19.6419, -15.2653) (19.6359, -15.2533) (19.6899, -15.0853) (19.7019, -15.0314) knots 70 70 70 70 71 71 71 71
  line L1246 (19.6419, -15.2653) -> (19.6359, -15.2533) construction
  line L1247 (19.6359, -15.2533) -> (19.6899, -15.0853) construction
  line L1248 (19.6899, -15.0853) -> (19.7019, -15.0314) construction
  spline S377 degree 3 poles (19.7019, -15.0314) (19.7319, -14.9113) (19.7619, -14.7913) (19.7979, -14.6713) knots 71 71 71 71 72 72 72 72
  line L1249 (19.7019, -15.0314) -> (19.7319, -14.9113) construction
  line L1250 (19.7319, -14.9113) -> (19.7619, -14.7913) construction
  line L1251 (19.7619, -14.7913) -> (19.7979, -14.6713) construction
  spline S378 degree 3 poles (19.7979, -14.6713) (19.8279, -14.5514) (19.8578, -14.4374) (19.8939, -14.3234) knots 72 72 72 72 73 73 73 73
  line L1252 (19.7979, -14.6713) -> (19.8279, -14.5514) construction
  line L1253 (19.8279, -14.5514) -> (19.8578, -14.4374) construction
  line L1254 (19.8578, -14.4374) -> (19.8939, -14.3234) construction
  spline S379 degree 3 poles (19.8939, -14.3234) (19.9238, -14.2154) (19.9659, -14.1614) (20.0319, -14.0774) knots 73 73 73 73 74 74 74 74
  line L1255 (19.8939, -14.3234) -> (19.9238, -14.2154) construction
  line L1256 (19.9238, -14.2154) -> (19.9659, -14.1614) construction
  line L1257 (19.9659, -14.1614) -> (20.0319, -14.0774) construction
  spline S380 degree 3 poles (20.0319, -14.0774) (20.3018, -13.7414) (20.5479, -13.3754) (20.7758, -13.0094) knots 74 74 74 74 75 75 75 75
  line L1258 (20.0319, -14.0774) -> (20.3018, -13.7414) construction
  line L1259 (20.3018, -13.7414) -> (20.5479, -13.3754) construction
  line L1260 (20.5479, -13.3754) -> (20.7758, -13.0094) construction
  spline S381 degree 3 poles (20.7758, -13.0094) (20.8598, -12.8714) (20.9138, -12.7514) (21.0158, -12.6374) knots 75 75 75 75 76 76 76 76
  line L1261 (20.7758, -13.0094) -> (20.8598, -12.8714) construction
  line L1262 (20.8598, -12.8714) -> (20.9138, -12.7514) construction
  line L1263 (20.9138, -12.7514) -> (21.0158, -12.6374) construction
  spline S382 degree 3 poles (21.0158, -12.6374) (21.1658, -12.4814) (21.2691, -12.2474) (21.3651, -12.0554) knots 76 76 76 76 77 77 77 77
  line L1264 (21.0158, -12.6374) -> (21.1658, -12.4814) construction
  line L1265 (21.1658, -12.4814) -> (21.2691, -12.2474) construction
  line L1266 (21.2691, -12.2474) -> (21.3651, -12.0554) construction
  spline S383 degree 3 poles (21.3651, -12.0554) (21.5271, -11.7434) (21.75, -11.3114) (21.7083, -10.9454) knots 77 77 77 77 78 78 78 78
  line L1267 (21.3651, -12.0554) -> (21.5271, -11.7434) construction
  line L1268 (21.5271, -11.7434) -> (21.75, -11.3114) construction
  line L1269 (21.75, -11.3114) -> (21.7083, -10.9454) construction
  line L1270 (21.7083, -10.9454) -> (21.7083, -10.9154)
  line L1271 (21.7083, -10.9154) -> (21.7011, -10.9094)
  spline S384 degree 3 poles (21.7011, -10.9094) (21.6651, -10.6754) (21.4485, -10.3994) (21.1845, -10.4834) knots 80 80 80 80 81 81 81 81
  line L1272 (21.7011, -10.9094) -> (21.6651, -10.6754) construction
  line L1273 (21.6651, -10.6754) -> (21.4485, -10.3994) construction
  line L1274 (21.4485, -10.3994) -> (21.1845, -10.4834) construction
  spline S385 degree 3 poles (21.1845, -10.4834) (21.0465, -10.5254) (20.9441, -10.6694) (20.8601, -10.7714) knots 81 81 81 81 82 82 82 82
  line L1275 (21.1845, -10.4834) -> (21.0465, -10.5254) construction
  line L1276 (21.0465, -10.5254) -> (20.9441, -10.6694) construction
  line L1277 (20.9441, -10.6694) -> (20.8601, -10.7714) construction
  line L1278 (20.8601, -10.7714) -> (20.722, -10.9574)
  spline S386 degree 3 poles (20.722, -10.9574) (20.692, -10.9934) (20.6499, -11.0834) (20.6199, -11.1314) knots 83 83 83 83 84 84 84 84
  line L1279 (20.722, -10.9574) -> (20.692, -10.9934) construction
  line L1280 (20.692, -10.9934) -> (20.6499, -11.0834) construction
  line L1281 (20.6499, -11.0834) -> (20.6199, -11.1314) construction
  line L1282 (20.6199, -11.1314) -> (20.6259, -11.1254)
  line L1283 (20.6259, -11.1254) -> (20.4339, -11.4554)
  line L1284 (20.4339, -11.4554) -> (20.4819, -11.3534)
  spline S387 degree 3 poles (20.4819, -11.3534) (20.4519, -11.3474) (20.3198, -11.6054) (20.3018, -11.6354) knots 87 87 87 87 88 88 88 88
  line L1285 (20.4819, -11.3534) -> (20.4519, -11.3474) construction
  line L1286 (20.4519, -11.3474) -> (20.3198, -11.6054) construction
  line L1287 (20.3198, -11.6054) -> (20.3018, -11.6354) construction
  spline S388 degree 3 poles (20.3018, -11.6354) (20.2359, -11.7494) (20.1758, -11.8634) (20.1218, -11.9774) knots 88 88 88 88 89 89 89 89
  line L1288 (20.3018, -11.6354) -> (20.2359, -11.7494) construction
  line L1289 (20.2359, -11.7494) -> (20.1758, -11.8634) construction
  line L1290 (20.1758, -11.8634) -> (20.1218, -11.9774) construction
  spline S389 degree 3 poles (20.1218, -11.9774) (20.0019, -12.2174) (19.8819, -12.4634) (19.8039, -12.7214) knots 89 89 89 89 90 90 90 90
  line L1291 (20.1218, -11.9774) -> (20.0019, -12.2174) construction
  line L1292 (20.0019, -12.2174) -> (19.8819, -12.4634) construction
  line L1293 (19.8819, -12.4634) -> (19.8039, -12.7214) construction
  spline S390 degree 3 poles (19.8039, -12.7214) (19.7199, -12.9794) (19.6239, -13.2314) (19.5339, -13.4894) knots 90 90 90 90 91 91 91 91
  line L1294 (19.8039, -12.7214) -> (19.7199, -12.9794) construction
  line L1295 (19.7199, -12.9794) -> (19.6239, -13.2314) construction
  line L1296 (19.6239, -13.2314) -> (19.5339, -13.4894) construction
  spline S391 degree 3 poles (19.5339, -13.4894) (19.4859, -13.6274) (19.4379, -13.7734) (19.3959, -13.9113) knots 91 91 91 91 92 92 92 92
  line L1297 (19.5339, -13.4894) -> (19.4859, -13.6274) construction
  line L1298 (19.4859, -13.6274) -> (19.4379, -13.7734) construction
  line L1299 (19.4379, -13.7734) -> (19.3959, -13.9113) construction
  spline S392 degree 3 poles (19.3959, -13.9113) (19.3599, -14.0253) (19.2759, -14.2083) (19.2939, -14.3333) knots 92 92 92 92 93 93 93 93
  line L1300 (19.3959, -13.9113) -> (19.3599, -14.0253) construction
  line L1301 (19.3599, -14.0253) -> (19.2759, -14.2083) construction
  line L1302 (19.2759, -14.2083) -> (19.2939, -14.3333) construction
  line L1303 (19.2939, -14.3333) -> (19.3119, -14.3333)
  spline S393 degree 3 poles (19.3119, -14.3333) (19.2939, -14.375) (19.2819, -14.4153) (19.2699, -14.4574) knots 94 94 94 94 95 95 95 95
  line L1304 (19.3119, -14.3333) -> (19.2939, -14.375) construction
  line L1305 (19.2939, -14.375) -> (19.2819, -14.4153) construction
  line L1306 (19.2819, -14.4153) -> (19.2699, -14.4574) construction
  spline S394 degree 3 poles (19.2699, -14.4574) (19.2759, -14.4213) (19.2759, -14.3784) (19.2819, -14.3664) knots 95 95 95 95 96 96 96 96
  line L1307 (19.2699, -14.4574) -> (19.2759, -14.4213) construction
  line L1308 (19.2759, -14.4213) -> (19.2759, -14.3784) construction
  line L1309 (19.2759, -14.3784) -> (19.2819, -14.3664) construction
  spline S395 degree 3 poles (19.2819, -14.3664) (19.2519, -14.4083) (19.2579, -14.5518) (19.2519, -14.5638) knots 96 96 96 96 97 97 97 97
  line L1310 (19.2819, -14.3664) -> (19.2519, -14.4083) construction
  line L1311 (19.2519, -14.4083) -> (19.2579, -14.5518) construction
  line L1312 (19.2579, -14.5518) -> (19.2519, -14.5638) construction
  spline S396 degree 3 poles (19.2519, -14.5638) (19.1739, -14.8878) (19.0839, -15.2116) (19.0599, -15.5476) knots 97 97 97 97 98 98 98 98
  line L1313 (19.2519, -14.5638) -> (19.1739, -14.8878) construction
  line L1314 (19.1739, -14.8878) -> (19.0839, -15.2116) construction
  line L1315 (19.0839, -15.2116) -> (19.0599, -15.5476) construction
  spline S397 degree 3 poles (19.0599, -15.5476) (19.0419, -15.8656) (19.0419, -16.2854) (19.2939, -16.5194) knots 98 98 98 98 99 99 99 99
  line L1316 (19.0599, -15.5476) -> (19.0419, -15.8656) construction
  line L1317 (19.0419, -15.8656) -> (19.0419, -16.2854) construction
  line L1318 (19.0419, -16.2854) -> (19.2939, -16.5194) construction
  spline S398 degree 3 poles (19.2939, -16.5194) (19.5759, -16.7774) (19.8999, -16.6034) (20.1339, -16.3814) knots 99 99 99 99 100 100 100 100
  line L1319 (19.2939, -16.5194) -> (19.5759, -16.7774) construction
  line L1320 (19.5759, -16.7774) -> (19.8999, -16.6034) construction
  line L1321 (19.8999, -16.6034) -> (20.1339, -16.3814) construction
  spline S399 degree 3 poles (20.1339, -16.3814) (20.4099, -16.1114) (20.6438, -15.7934) (20.8598, -15.4814) knots 100 100 100 100 101 101 101 101
  line L1322 (20.1339, -16.3814) -> (20.4099, -16.1114) construction
  line L1323 (20.4099, -16.1114) -> (20.6438, -15.7934) construction
  line L1324 (20.6438, -15.7934) -> (20.8598, -15.4814) construction
  spline S400 degree 3 poles (20.8598, -15.4814) (20.9818, -15.304) (21.0877, -15.1199) (21.1932, -14.9373) knots 101 101 101 101 102 102 102 102
  line L1325 (20.8598, -15.4814) -> (20.9818, -15.304) construction
  line L1326 (20.9818, -15.304) -> (21.0877, -15.1199) construction
  line L1327 (21.0877, -15.1199) -> (21.1932, -14.9373) construction
  spline S401 degree 3 poles (21.1932, -14.9373) (21.2426, -15.1771) (21.4049, -15.3987) (21.6218, -15.5053) knots 102 102 102 102 103 103 103 103
  line L1328 (21.1932, -14.9373) -> (21.2426, -15.1771) construction
  line L1329 (21.2426, -15.1771) -> (21.4049, -15.3987) construction
  line L1330 (21.4049, -15.3987) -> (21.6218, -15.5053) construction
  spline S402 degree 3 poles (21.6218, -15.5053) (21.7358, -15.5593) (21.8678, -15.5833) (21.9878, -15.5713) knots 103 103 103 103 104 104 104 104
  line L1331 (21.6218, -15.5053) -> (21.7358, -15.5593) construction
  line L1332 (21.7358, -15.5593) -> (21.8678, -15.5833) construction
  line L1333 (21.8678, -15.5833) -> (21.9878, -15.5713) construction
  spline S403 degree 3 poles (21.9878, -15.5713) (22.1138, -15.5533) (22.2338, -15.4873) (22.3298, -15.4153) knots 104 104 104 104 105 105 105 105
  line L1334 (21.9878, -15.5713) -> (22.1138, -15.5533) construction
  line L1335 (22.1138, -15.5533) -> (22.2338, -15.4873) construction
  line L1336 (22.2338, -15.4873) -> (22.3298, -15.4153) construction
  spline S404 degree 3 poles (22.3298, -15.4153) (22.4198, -15.3493) (22.6178, -15.2293) (22.6538, -15.1273) knots 105 105 105 105 106 106 106 106
  line L1337 (22.3298, -15.4153) -> (22.4198, -15.3493) construction
  line L1338 (22.4198, -15.3493) -> (22.6178, -15.2293) construction
  line L1339 (22.6178, -15.2293) -> (22.6538, -15.1273) construction
  spline S405 degree 3 poles (22.6538, -15.1273) (22.6538, -15.1213) (22.6418, -15.1273) (22.6238, -15.1453) knots 106 106 106 106 107 107 107 107
  line L1340 (22.6538, -15.1273) -> (22.6538, -15.1213) construction
  line L1341 (22.6538, -15.1213) -> (22.6418, -15.1273) construction
  line L1342 (22.6418, -15.1273) -> (22.6238, -15.1453) construction
  line L1343 (22.6238, -15.1453) -> (22.7978, -14.9413)
  spline S406 degree 3 poles (22.7978, -14.9413) (22.8038, -14.9473) (22.7558, -15.0073) (22.7558, -15.0073) knots 108 108 108 108 109 109 109 109
  line L1344 (22.7978, -14.9413) -> (22.8038, -14.9473) construction
  line L1345 (22.8038, -14.9473) -> (22.7558, -15.0073) construction
  line L1346 (22.7558, -15.0073) -> (22.7558, -15.0073) construction
  spline S407 degree 3 poles (22.7558, -15.0073) (22.7978, -15.0253) (23.0138, -14.7074) (23.0378, -14.6833) knots 109 109 109 109 110 110 110 110